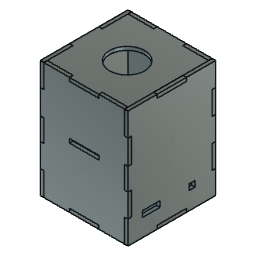
Project1box (Autodesk Fusion 360 design; units mm, degrees)
Autodesk Fusion 360 part; units mm, degrees
sketch "base" plane through (0, 0, 0) normal (0, 0, 1) x (1, 0, 0)
  line L0 (0, 2.6463) -> (75, 2.6463)
  line L1 (75, 2.6463) -> (75, 77.6463)
  line L2 (75, 77.6463) -> (0, 77.6463)
  line L3 (0, 77.6463) -> (0, 2.6463)
  dimension "d8" = 75
  dimension "d9" = 75
  constraint horizontal L0
  constraint vertical L1
  constraint horizontal L2
  constraint vertical L3
  measures "d8" distance of L0.start L2.end
  measures "d9" distance of L0.start L0.end
extrude "Extrude1" add sketch "base" along normal blind 3 makes body 1
sketch "front" plane through (0, 2.6463, 0) normal (0, -1, 0) x (1, 0, 0)
  line L0 (0, 0) -> (75, 0)
  line L1 (75, 0) -> (75, 3)
  line L2 (75, 3) -> (0, 3)
  line L3 (0, 3) -> (0, 0)
  line L4 (0, 0) -> (75, 0)
  line L5 (75, 0) -> (75, 100)
  line L6 (75, 100) -> (0, 100)
  line L7 (0, 100) -> (0, 0)
  line L8 (25, 0) -> (50, 0)
  line L9 (50, 0) -> (50, 3)
  line L10 (50, 3) -> (25, 3)
  line L11 (25, 3) -> (25, 0)
  dimension "d16" = 100
  dimension "d21" = 25
  dimension "d22" = 25
  dimension "d23" = 25
  constraint perpendicular L4 L5
  constraint parallel L4 L6
  constraint parallel L5 L7
  constraint coincident L0.end L1.start
  constraint perpendicular L1 L4
  constraint coincident L0.start L3.end
  constraint perpendicular L8 L9
  constraint parallel L8 L10
  constraint parallel L9 L11
  constraint coincident L4 L8.end
  constraint parallel L4 L8
  measures "d16" distance of L0.start L6.end
  measures "d21" distance of L0.start L8.start
  measures "d22" distance of L8.start L8.end
  measures "d23" distance of L0.end L8.end
extrude "Extrude2" add sketch "front" against normal blind 3 separate body contours L0 L2 L3 L4 L7 L11 | L2 L5 L6 L7 L10 | L0 L1 L2 L4 L5 L9 makes body 2
extrude "Extrude3" add 1 faces at (33.3333, 5.6463, 67.6667) along direction (0, -1, 0) blind 3 from surface at -72 separate body on bodies 2 makes body 3
combine "Combine1" operation cut target body 1 tool bodies 3 2 keep tools
sketch "Sketch6" plane through (0, 0, 0) normal (1, 0, 0) x (0, 1, 0)
  line L0 (2.6463, 100) -> (2.6463, 0)
  line L1 (2.6463, 0) -> (5.6463, 0)
  line L2 (5.6463, 0) -> (5.6463, 100)
  line L3 (5.6463, 100) -> (2.6463, 100)
  line L4 (77.6463, 0) -> (77.6463, 100)
  line L5 (77.6463, 100) -> (74.6463, 100)
  line L6 (74.6463, 100) -> (74.6463, 0)
  line L7 (74.6463, 0) -> (77.6463, 0)
  line L8 (27.6463, 0) -> (52.6463, 0)
  line L9 (52.6463, 0) -> (52.6463, 3)
  line L10 (52.6463, 3) -> (27.6463, 3)
  line L11 (27.6463, 3) -> (27.6463, 0)
  line L12 (2.6463, 80) -> (5.6463, 80)
  line L13 (5.6463, 80) -> (5.6463, 60)
  line L14 (5.6463, 60) -> (2.6463, 60)
  line L15 (2.6463, 60) -> (2.6463, 80)
  line L16 (2.6463, 59.0388) -> (2.6463, 40)
  line L17 (2.6463, 40) -> (5.6463, 40)
  line L18 (5.6463, 40) -> (5.6463, 59.0388)
  line L19 (5.6463, 59.0388) -> (2.6463, 59.0388)
  line L20 (2.6463, 39.2994) -> (2.6463, 20)
  line L21 (2.6463, 20) -> (5.6463, 20)
  line L22 (5.6463, 20) -> (5.6463, 39.2994)
  line L23 (5.6463, 39.2994) -> (2.6463, 39.2994)
  line L24 (74.6463, 80) -> (77.6463, 80)
  line L25 (77.6463, 80) -> (77.6463, 63.0399)
  line L26 (77.6463, 63.0399) -> (74.6463, 63.0399)
  line L27 (74.6463, 63.0399) -> (74.6463, 80)
  line L28 (74.6463, 60) -> (77.6463, 60)
  line L29 (77.6463, 60) -> (77.6463, 40)
  line L30 (77.6463, 40) -> (74.6463, 40)
  line L31 (74.6463, 40) -> (74.6463, 60)
  line L32 (74.6463, 38.1297) -> (77.6463, 38.1297)
  line L33 (77.6463, 38.1297) -> (77.6463, 20)
  line L34 (77.6463, 20) -> (74.6463, 20)
  line L35 (74.6463, 20) -> (74.6463, 38.1297)
  line L36 (2.6463, 0) -> (77.6463, 0)
  line L37 (77.6463, 0) -> (77.6463, 100)
  line L38 (77.6463, 100) -> (2.6463, 100)
  line L39 (2.6463, 100) -> (2.6463, 0)
  dimension "d29" = 3
  dimension "d30" = 25
  dimension "d31" = 25
  dimension "d32" = 25
  dimension "d33" = 20
  dimension "d34" = 20
  dimension "d35" = 20
  dimension "d36" = 20
  dimension "d37" = 20
  dimension "d38" = 20
  dimension "d39" = 20
  dimension "d40" = 20
  dimension "d41" = 20
  dimension "d42" = 20
  constraint horizontal L8
  constraint vertical L9
  constraint horizontal L10
  constraint vertical L11
  constraint perpendicular L12 L13
  constraint parallel L12 L14
  constraint parallel L13 L15
  constraint coincident L2 L12.end
  constraint perpendicular L2 L12
  constraint coincident L0 L12.start
  constraint perpendicular L16 L17
  constraint parallel L16 L18
  constraint parallel L17 L19
  constraint coincident L0 L16.end
  constraint perpendicular L14 L16
  constraint perpendicular L20 L21
  constraint parallel L20 L22
  constraint parallel L21 L23
  constraint coincident L0 L20.end
  constraint perpendicular L19 L20
  constraint perpendicular L24 L25
  constraint parallel L24 L26
  constraint parallel L25 L27
  constraint coincident L4 L24.end
  constraint perpendicular L4 L24
  constraint coincident L6 L24.start
  constraint perpendicular L28 L29
  constraint parallel L28 L30
  constraint parallel L29 L31
  constraint coincident L4 L28.end
  constraint perpendicular L4 L28
  constraint coincident L6 L28.start
  constraint perpendicular L32 L33
  constraint parallel L32 L34
  constraint parallel L33 L35
  constraint coincident L4 L32.end
  constraint perpendicular L4 L32
  constraint coincident L6 L32.start
  constraint horizontal L36
  constraint vertical L37
  constraint horizontal L38
  constraint vertical L39
  constraint coincident L4.end L5.start
  constraint coincident L0.end L1.start
  measures "d29" distance of L8.start L10.end
  measures "d30" distance of L0.end L8.start
  measures "d31" distance of L8.start L8.end
  measures "d32" distance of L4.start L8.end
  measures "d33" distance of L0.start L12.start
  measures "d34" distance of L12.start L14.end
  measures "d35" distance of L14.end L16.end
  measures "d36" distance of L16.end L20.end
  measures "d37" distance of L0.end L20.end
  measures "d38" distance of L4.end L24.end
  measures "d39" distance of L24.end L28.end
  measures "d40" distance of L28.end L29.end
  measures "d41" distance of L29.end L33.end
  measures "d42" distance of L4.start L33.end
extrude "Extrude4" add sketch "Sketch6" along normal blind 3 separate body contours L0 L2 L3 L12 L38 L39 | L2 L6 L9 L10 L11 L13 L18 L22 L27 L31 L35 L36 L38 | L4 L5 L6 L24 L37 L38 | L0 L2 L16 L17 L18 L19 L39 | L4 L6 L28 L29 L30 L31 L37 | L0 L1 L2 L21 L36 L39 | L4 L6 L7 L34 L36 L37 makes body 4
extrude "Extrude6" add 1 faces at (3, 35.9796, 26.8097) along direction (-1, 0, 0) blind 3 from surface at -72 separate body on bodies 4 makes body 5
combine "Combine2" operation cut target body 2 tool bodies 4 5 keep tools
combine "Combine3" operation cut target body 3 tool bodies 4 5 keep tools
extrude "Extrude7" add 1 faces at (3, 35.9796, 26.8097) along direction (-1, 0, 0) blind 3 from surface at -72 on bodies 4 bodies 4 makes body 6
combine "Combine4" operation cut target body 1 tool bodies 4 6 keep tools
extrude "Extrude8" add 1 faces at (41.6667, 51.6463, 3) along direction (0, 0, -1) blind 3 from surface at -97 on bodies 1 bodies 1 makes body 7
combine "Combine5" operation cut target body 3 tool bodies 7 keep tools
combine "Combine6" operation cut target body 4 tool bodies 7 keep tools
combine "Combine7" operation cut target body 2 tool bodies 7 keep tools
combine "Combine8" operation cut target body 5 tool bodies 7 keep tools
sketch "Sketch7" plane through (0, 2.6463, 0) normal (0, -1, 0) x (1, 0, 0)
  line L0 (25, 97) -> (25, 100)
  line L1 (25, 100) -> (3, 100)
  line L2 (3, 100) -> (3, 80)
  line L3 (3, 80) -> (0, 80)
  line L4 (0, 80) -> (0, 59.0388)
  line L5 (0, 59.0388) -> (3, 59.0388)
  line L6 (3, 59.0388) -> (3, 40)
  line L7 (3, 40) -> (0, 40)
  line L8 (0, 40) -> (0, 20)
  line L9 (0, 20) -> (3, 20)
  line L10 (3, 20) -> (3, 0)
  line L11 (3, 0) -> (25, 0)
  line L12 (25, 0) -> (25, 3)
  line L13 (25, 3) -> (50, 3)
  line L14 (50, 3) -> (50, 0)
  line L15 (50, 0) -> (72, 0)
  line L16 (72, 0) -> (72, 20)
  line L17 (72, 20) -> (75, 20)
  line L18 (75, 20) -> (75, 40)
  line L19 (75, 40) -> (72, 40)
  line L20 (72, 40) -> (72, 59.0388)
  line L21 (72, 59.0388) -> (75, 59.0388)
  line L22 (75, 59.0388) -> (75, 80)
  line L23 (75, 80) -> (72, 80)
  line L24 (72, 80) -> (72, 100)
  line L25 (72, 100) -> (50, 100)
  line L26 (50, 100) -> (50, 97)
  line L27 (50, 97) -> (25, 97)
  line L28 (25, 54.7848) -> (50.2211, 54.7848)
  line L29 (50.2211, 54.7848) -> (50.2211, 51.2848)
  line L30 (50.2211, 51.2848) -> (25, 51.2848)
  line L31 (25, 51.2848) -> (25, 54.7848)
  dimension "d57" = 3.5
  dimension "d65" = 25.2211
  constraint horizontal L28
  constraint vertical L29
  constraint horizontal L30
  constraint vertical L31
  measures "d57" distance of L28.start L30.end
  measures "d65" distance of L28.start L28.end
extrude "Extrude9" cut sketch "Sketch7" against normal blind 130 contours L28 L29 L30 L31 bodies 2 3
sketch "Sketch8" plane through (0, 0, 100) normal (0, 0, 1) x (-1, 0, 0)
  line L0 (-75, -52.6463) -> (-72, -52.6463)
  line L1 (-72, -52.6463) -> (-72, -74.6463)
  line L2 (-72, -74.6463) -> (-50, -74.6463)
  line L3 (-50, -74.6463) -> (-50, -77.6463)
  line L4 (-50, -77.6463) -> (-25, -77.6463)
  line L5 (-25, -77.6463) -> (-25, -74.6463)
  line L6 (-25, -74.6463) -> (-3, -74.6463)
  line L7 (-3, -74.6463) -> (-3, -52.6463)
  line L8 (-3, -52.6463) -> (0, -52.6463)
  line L9 (0, -52.6463) -> (0, -27.6463)
  line L10 (0, -27.6463) -> (-3, -27.6463)
  line L11 (-3, -27.6463) -> (-3, -5.6463)
  line L12 (-3, -5.6463) -> (-25, -5.6463)
  line L13 (-25, -5.6463) -> (-25, -2.6463)
  line L14 (-25, -2.6463) -> (-50, -2.6463)
  line L15 (-50, -2.6463) -> (-50, -5.6463)
  line L16 (-50, -5.6463) -> (-72, -5.6463)
  line L17 (-72, -5.6463) -> (-72, -27.6463)
  line L18 (-72, -27.6463) -> (-75, -27.6463)
  line L19 (-75, -27.6463) -> (-75, -52.6463)
  circle A0 centre (-37.2569, -39.6601) radius 15
  dimension "d60" = 30
  measures "d60" diameter of A0
extrude "Extrude10" cut sketch "Sketch8" against normal blind 10 contours A0 bodies 7
sketch "Sketch9" plane through (0, 0, 0) normal (-1, 0, 0) x (0, -1, 0)
  line L0 (-27.6463, 100) -> (-27.6463, 97)
  line L1 (-27.6463, 97) -> (-52.6463, 97)
  line L2 (-52.6463, 97) -> (-52.6463, 100)
  line L3 (-52.6463, 100) -> (-77.6463, 100)
  line L4 (-77.6463, 100) -> (-77.6463, 80)
  line L5 (-77.6463, 80) -> (-74.6463, 80)
  line L6 (-74.6463, 80) -> (-74.6463, 60)
  line L7 (-74.6463, 60) -> (-77.6463, 60)
  line L8 (-77.6463, 60) -> (-77.6463, 40)
  line L9 (-77.6463, 40) -> (-74.6463, 40)
  line L10 (-74.6463, 40) -> (-74.6463, 20)
  line L11 (-74.6463, 20) -> (-77.6463, 20)
  line L12 (-77.6463, 20) -> (-77.6463, 0)
  line L13 (-77.6463, 0) -> (-52.6463, 0)
  line L14 (-52.6463, 0) -> (-52.6463, 3)
  line L15 (-52.6463, 3) -> (-27.6463, 3)
  line L16 (-27.6463, 3) -> (-27.6463, 0)
  line L17 (-27.6463, 0) -> (-2.6463, 0)
  line L18 (-2.6463, 0) -> (-2.6463, 20)
  line L19 (-2.6463, 20) -> (-5.6463, 20)
  line L20 (-5.6463, 20) -> (-5.6463, 40)
  line L21 (-5.6463, 40) -> (-2.6463, 40)
  line L22 (-2.6463, 40) -> (-2.6463, 59.0388)
  line L23 (-2.6463, 59.0388) -> (-5.6463, 59.0388)
  line L24 (-5.6463, 59.0388) -> (-5.6463, 80)
  line L25 (-5.6463, 80) -> (-2.6463, 80)
  line L26 (-2.6463, 80) -> (-2.6463, 100)
  line L27 (-2.6463, 100) -> (-27.6463, 100)
sketch "Sketch10" plane through (75, 0, 0) normal (1, 0, 0) x (0, 1, 0)
  line L0 (77.6463, 60) -> (74.6463, 60)
  line L1 (74.6463, 60) -> (74.6463, 80)
  line L2 (74.6463, 80) -> (77.6463, 80)
  line L3 (77.6463, 80) -> (77.6463, 100)
  line L4 (77.6463, 100) -> (2.6463, 100)
  line L5 (2.6463, 100) -> (2.6463, 80)
  line L6 (2.6463, 80) -> (5.6463, 80)
  line L7 (5.6463, 80) -> (5.6463, 59.0388)
  line L8 (5.6463, 59.0388) -> (2.6463, 59.0388)
  line L9 (2.6463, 59.0388) -> (2.6463, 40)
  line L10 (2.6463, 40) -> (5.6463, 40)
  line L11 (5.6463, 40) -> (5.6463, 20)
  line L12 (5.6463, 20) -> (2.6463, 20)
  line L13 (2.6463, 20) -> (2.6463, 0)
  line L14 (2.6463, 0) -> (27.6463, 0)
  line L15 (27.6463, 0) -> (27.6463, 3)
  line L16 (27.6463, 3) -> (52.6463, 3)
  line L17 (52.6463, 3) -> (52.6463, 0)
  line L18 (52.6463, 0) -> (77.6463, 0)
  line L19 (77.6463, 0) -> (77.6463, 20)
  line L20 (77.6463, 20) -> (74.6463, 20)
  line L21 (74.6463, 20) -> (74.6463, 40)
  line L22 (74.6463, 40) -> (77.6463, 40)
  line L23 (77.6463, 40) -> (77.6463, 60)
  line L24 (15, 20) -> (30, 20)
  line L25 (30, 20) -> (30, 15)
  line L26 (30, 15) -> (15, 15)
  line L27 (15, 15) -> (15, 20)
  line L28 (55, 20) -> (60, 20)
  line L29 (60, 20) -> (60, 15)
  line L30 (60, 15) -> (55, 15)
  line L31 (55, 15) -> (55, 20)
  constraint horizontal L24
  constraint vertical L25
  constraint horizontal L26
  constraint vertical L27
  constraint horizontal L28
  constraint vertical L29
  constraint horizontal L30
  constraint vertical L31
extrude "Extrude11" cut sketch "Sketch10" against normal blind 15 contours L24 L25 L26 L27 | L28 L29 L30 L31 bodies 5 6
sketch "Sketch12" plane through (0, 2.6463, 0) normal (0, -1, 0) x (1, 0, 0)
  line L0 (50.2211, 54.7848) -> (50.2211, 51.2848)
  line L1 (50.2211, 51.2848) -> (25, 51.2848)
  line L2 (25, 51.2848) -> (25, 54.7848)
  line L3 (25, 54.7848) -> (50.2211, 54.7848)
  line L4 (25, 97) -> (25, 100)
  line L5 (25, 100) -> (3, 100)
  line L6 (3, 100) -> (3, 80)
  line L7 (3, 80) -> (0, 80)
  line L8 (0, 80) -> (0, 59.0388)
  line L9 (0, 59.0388) -> (3, 59.0388)
  line L10 (3, 59.0388) -> (3, 40)
  line L11 (3, 40) -> (0, 40)
  line L12 (0, 40) -> (0, 20)
  line L13 (0, 20) -> (3, 20)
  line L14 (3, 20) -> (3, 0)
  line L15 (3, 0) -> (25, 0)
  line L16 (25, 0) -> (25, 3)
  line L17 (25, 3) -> (50, 3)
  line L18 (50, 3) -> (50, 0)
  line L19 (50, 0) -> (72, 0)
  line L20 (72, 0) -> (72, 20)
  line L21 (72, 20) -> (75, 20)
  line L22 (75, 20) -> (75, 40)
  line L23 (75, 40) -> (72, 40)
  line L24 (72, 40) -> (72, 59.0388)
  line L25 (72, 59.0388) -> (75, 59.0388)
  line L26 (75, 59.0388) -> (75, 80)
  line L27 (75, 80) -> (72, 80)
  line L28 (72, 80) -> (72, 100)
  line L29 (72, 100) -> (50, 100)
  line L30 (50, 100) -> (50, 97)
  line L31 (50, 97) -> (25, 97)
sketch "Sketch13" plane through (75, 0, 0) normal (1, 0, 0) x (0, 1, 0)
  line L0 (30, 20) -> (30, 15)
  line L1 (30, 15) -> (15, 15)
  line L2 (15, 15) -> (15, 20)
  line L3 (15, 20) -> (30, 20)
  line L4 (60, 20) -> (60, 15)
  line L5 (60, 15) -> (55, 15)
  line L6 (55, 15) -> (55, 20)
  line L7 (55, 20) -> (60, 20)
  line L8 (52.6463, 100) -> (52.6463, 97)
  line L9 (52.6463, 97) -> (27.6463, 97)
  line L10 (27.6463, 97) -> (27.6463, 100)
  line L11 (27.6463, 100) -> (2.6463, 100)
  line L12 (2.6463, 100) -> (2.6463, 80)
  line L13 (2.6463, 80) -> (5.6463, 80)
  line L14 (5.6463, 80) -> (5.6463, 59.0388)
  line L15 (5.6463, 59.0388) -> (2.6463, 59.0388)
  line L16 (2.6463, 59.0388) -> (2.6463, 40)
  line L17 (2.6463, 40) -> (5.6463, 40)
  line L18 (5.6463, 40) -> (5.6463, 20)
  line L19 (5.6463, 20) -> (2.6463, 20)
  line L20 (2.6463, 20) -> (2.6463, 0)
  line L21 (2.6463, 0) -> (27.6463, 0)
  line L22 (27.6463, 0) -> (27.6463, 3)
  line L23 (27.6463, 3) -> (52.6463, 3)
  line L24 (52.6463, 3) -> (52.6463, 0)
  line L25 (52.6463, 0) -> (77.6463, 0)
  line L26 (77.6463, 0) -> (77.6463, 20)
  line L27 (77.6463, 20) -> (74.6463, 20)
  line L28 (74.6463, 20) -> (74.6463, 40)
  line L29 (74.6463, 40) -> (77.6463, 40)
  line L30 (77.6463, 40) -> (77.6463, 60)
  line L31 (77.6463, 60) -> (74.6463, 60)
  line L32 (74.6463, 60) -> (74.6463, 80)
  line L33 (74.6463, 80) -> (77.6463, 80)
  line L34 (77.6463, 80) -> (77.6463, 100)
  line L35 (77.6463, 100) -> (52.6463, 100)
sketch "Sketch14" plane through (0, 77.6463, 0) normal (0, 1, 0) x (-1, 0, 0)
  line L0 (-50.2211, 51.2848) -> (-50.2211, 54.7848)
  line L1 (-50.2211, 54.7848) -> (-25, 54.7848)
  line L2 (-25, 54.7848) -> (-25, 51.2848)
  line L3 (-25, 51.2848) -> (-50.2211, 51.2848)
  line L4 (-50, 97) -> (-50, 100)
  line L5 (-50, 100) -> (-72, 100)
  line L6 (-72, 100) -> (-72, 80)
  line L7 (-72, 80) -> (-75, 80)
  line L8 (-75, 80) -> (-75, 60)
  line L9 (-75, 60) -> (-72, 60)
  line L10 (-72, 60) -> (-72, 40)
  line L11 (-72, 40) -> (-75, 40)
  line L12 (-75, 40) -> (-75, 20)
  line L13 (-75, 20) -> (-72, 20)
  line L14 (-72, 20) -> (-72, 0)
  line L15 (-72, 0) -> (-50, 0)
  line L16 (-50, 0) -> (-50, 3)
  line L17 (-50, 3) -> (-25, 3)
  line L18 (-25, 3) -> (-25, 0)
  line L19 (-25, 0) -> (-3, 0)
  line L20 (-3, 0) -> (-3, 20)
  line L21 (-3, 20) -> (0, 20)
  line L22 (0, 20) -> (0, 40)
  line L23 (0, 40) -> (-3, 40)
  line L24 (-3, 40) -> (-3, 60)
  line L25 (-3, 60) -> (0, 60)
  line L26 (0, 60) -> (0, 80)
  line L27 (0, 80) -> (-3, 80)
  line L28 (-3, 80) -> (-3, 100)
  line L29 (-3, 100) -> (-25, 100)
  line L30 (-25, 100) -> (-25, 97)
  line L31 (-25, 97) -> (-50, 97)
sketch "Sketch16" plane through (0, 0, 100) normal (0, 0, 1) x (-1, 0, 0)
  circle A0 centre (-37.2569, -39.6601) radius 15
  line L0 (-75, -52.6463) -> (-72, -52.6463)
  line L1 (-72, -52.6463) -> (-72, -74.6463)
  line L2 (-72, -74.6463) -> (-50, -74.6463)
  line L3 (-50, -74.6463) -> (-50, -77.6463)
  line L4 (-50, -77.6463) -> (-25, -77.6463)
  line L5 (-25, -77.6463) -> (-25, -74.6463)
  line L6 (-25, -74.6463) -> (-3, -74.6463)
  line L7 (-3, -74.6463) -> (-3, -52.6463)
  line L8 (-3, -52.6463) -> (0, -52.6463)
  line L9 (0, -52.6463) -> (0, -27.6463)
  line L10 (0, -27.6463) -> (-3, -27.6463)
  line L11 (-3, -27.6463) -> (-3, -5.6463)
  line L12 (-3, -5.6463) -> (-25, -5.6463)
  line L13 (-25, -5.6463) -> (-25, -2.6463)
  line L14 (-25, -2.6463) -> (-50, -2.6463)
  line L15 (-50, -2.6463) -> (-50, -5.6463)
  line L16 (-50, -5.6463) -> (-72, -5.6463)
  line L17 (-72, -5.6463) -> (-72, -27.6463)
  line L18 (-72, -27.6463) -> (-75, -27.6463)
  line L19 (-75, -27.6463) -> (-75, -52.6463)
sketch "Sketch17" plane through (0, 0, 0) normal (0, 0, -1) x (1, 0, 0)
  line L0 (72, -74.6463) -> (72, -52.6463)
  line L1 (72, -52.6463) -> (75, -52.6463)
  line L2 (75, -52.6463) -> (75, -27.6463)
  line L3 (75, -27.6463) -> (72, -27.6463)
  line L4 (72, -27.6463) -> (72, -5.6463)
  line L5 (72, -5.6463) -> (50, -5.6463)
  line L6 (50, -5.6463) -> (50, -2.6463)
  line L7 (50, -2.6463) -> (25, -2.6463)
  line L8 (25, -2.6463) -> (25, -5.6463)
  line L9 (25, -5.6463) -> (3, -5.6463)
  line L10 (3, -5.6463) -> (3, -27.6463)
  line L11 (3, -27.6463) -> (0, -27.6463)
  line L12 (0, -27.6463) -> (0, -52.6463)
  line L13 (0, -52.6463) -> (3, -52.6463)
  line L14 (3, -52.6463) -> (3, -74.6463)
  line L15 (3, -74.6463) -> (25, -74.6463)
  line L16 (25, -74.6463) -> (25, -77.6463)
  line L17 (25, -77.6463) -> (50, -77.6463)
  line L18 (50, -77.6463) -> (50, -74.6463)
  line L19 (50, -74.6463) -> (72, -74.6463)
equation "length = 75 mm" comment "box length"
equation "width = 75 mm" comment "box width"
equation "height = 100 mm"
equation "hole = 60 mm"
equation "thickness = 3 mm"
equation "d8 = width"
equation "d9 = length"
equation "d10 = thickness"
equation "slotL = length / 3" comment "size of slot @length"
equation "slotW = width / 3" comment "size of slot@width"
equation "slotH = height / 5" comment "size of slot@height"
equation "d16 = height"
equation "d21 = slotL"
equation "d22 = slotL"
equation "d24 = -thickness"
equation "d27 = -thickness"
equation "d29 = thickness"
equation "d30 = slotW"
equation "d31 = slotW"
equation "d33 = slotH"
equation "d34 = slotH"
equation "d35 = slotH"
equation "d36 = slotH"
equation "d38 = slotH"
equation "d39 = slotH"
equation "d40 = slotH"
equation "d41 = slotH"
equation "d43 = thickness"
equation "d49 = -thickness"
equation "d52 = -thickness"
equation "d55 = -thickness"
named bodies: "Base", "Front", "Right", "Back"
